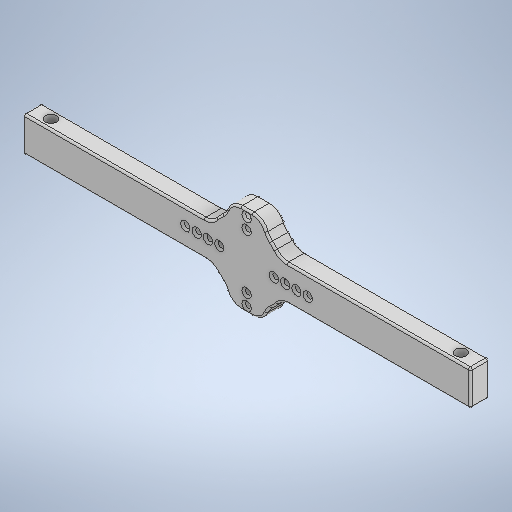
# Autodesk Inventor part: ServoAdapter
Saved by Autodesk Inventor 2025 (Build 290162000, 162)
## iProperties
Created: 2025-12-03
Part Number: ServoAdapter
Material: Generic
Document SubType Name: Modeling
Designer: ruven
Density: 1 g/cm^3
Appearance: Default
Author: ruven
Autodesk Inventor part; units mm, degrees
ref_plane "YZ Plane" through (0, 0, 0) normal (1, 0, 0) x (0, 1, 0)
ref_plane "XZ Plane" through (0, 0, 0) normal (0, 1, 0) x (-1, 0, 0)
ref_plane "XY Plane" through (0, 0, 0) normal (0, 0, 1) x (1, 0, 0)
sketch "Sketch1" plane through (0, 0, 0) normal (0, 1, 0) x (-1, 0, 0)
  line L0 (-59.4421, -4.3335) -> (-59.4421, 5)
  line L1 (59.4421, 4.3335) -> (59.4421, -5)
  line L2 (59.4421, -5) -> (-59.4421, 5) construction
  line L3 (-59.4421, -4.3335) -> (59.4421, 4.3335) construction
  line L4 (5, -59.443) -> (-5, -59.443)
  line L5 (-5, 59.443) -> (5, 59.443)
  line L6 (5, -59.443) -> (-5, 59.443) construction
  line L7 (-5, -59.443) -> (5, 59.443) construction
  circle A0 centre (0, 54.443) radius 2
  circle A1 centre (0, -54.443) radius 2
  line L8 (9.0122, 4.3335) -> (59.4421, 4.3335)
  line L9 (5, 18.5) -> (5, 8.6603)
  line L10 (5, 0.3645) -> (5, -0.4206)
  line L11 (5, -8.6603) -> (5, -18.5)
  line L12 (59.4421, -5) -> (8.6603, -5)
  line L13 (0.4206, -5) -> (-0.4206, -5)
  line L14 (-9.0122, -4.3335) -> (-59.4421, -4.3335)
  line L15 (-5, -18.5) -> (-5, -8.6603)
  line L16 (-5.0006, -0.3646) -> (-5.0006, 0.4206)
  line L17 (-5, 8.6603) -> (-5, 18.5)
  line L18 (-59.4421, 5) -> (-8.6603, 5)
  line L19 (-0.4206, 5) -> (0.4206, 5)
  circle A2 centre (0, 7.25) radius 0.75
  circle A3 centre (0, 10.25) radius 0.75
  circle A4 centre (0, 13.25) radius 0.75
  circle A5 centre (0, 16.25) radius 0.75
  line L20 (10.3146, 0) -> (-7.4821, 0) construction
  line L21 (0, -8.9076) -> (0, 6.1555) construction
  circle A6 centre (0, -7.25) radius 0.75
  circle A7 centre (0, -10.25) radius 0.75
  circle A8 centre (0, -13.25) radius 0.75
  circle A9 centre (0, -16.25) radius 0.75
  line L22 (59.443, -5) -> (-59.443, 5) construction
  line L23 (-5, -0.4206) -> (-5, 0.4206)
  circle A10 centre (-7.25, 0) radius 0.75
  circle A11 centre (-10.25, 0) radius 0.75
  circle A12 centre (-16.25, 0) radius 0.75
  circle A13 centre (-13.25, 0) radius 0.75
  line L24 (5, 0.4206) -> (5, -0.4206)
  circle A14 centre (7.25, 0) radius 0.75
  circle A15 centre (10.25, 0) radius 0.75
  circle A16 centre (13.25, 0) radius 0.75
  circle A17 centre (16.25, 0) radius 0.75
  line L25 (8.9076, 0) -> (-6.1555, 0) construction
  arc A18 (-0.7496, 10.2256) -> (-0.8594, 10.217) centre (0, 0) ccw
  arc A19 (0.8594, 10.217) -> (0.7496, 10.2256) centre (0, 0) ccw
  arc A20 (-5, 8.6603) -> (-8.6603, 5) centre (0, 0) ccw
  arc A21 (-10.217, 0.8594) -> (-10.2256, 0.7496) centre (0, 0) ccw
  arc A22 (-10.2258, -0.7496) -> (-10.2261, -0.7455) centre (0, 0) ccw
  arc A23 (-9.0122, -4.3335) -> (-5, -8.6603) centre (0, 0) ccw
  arc A24 (-0.8594, -10.217) -> (-0.7496, -10.2256) centre (0, 0) ccw
  arc A25 (0.7496, -10.2256) -> (0.8594, -10.217) centre (0, 0) ccw
  arc A26 (5, -8.6603) -> (8.6603, -5) centre (0, 0) ccw
  arc A27 (9.0122, 4.3335) -> (5, 8.6603) centre (0, 0) ccw
  arc A28 (10.217, -0.8594) -> (10.2256, -0.7496) centre (0, 0) ccw
  arc A29 (10.2532, 0) -> (10.2261, 0.7455) centre (0, 0) ccw
  line L26 (5, 18.5) -> (-5, 18.5)
  line L27 (-5, -18.5) -> (5, -18.5)
  point P0 (0, -59.443)
  point P1 (0, -6.1555)
  point P2 (6.1555, 0)
  point P3 (0, 0)
  dimension "d0" = 118.886
  dimension "d1" = 118.886
  dimension "d4" = 4
  dimension "d5" = 4
  dimension "d10" = 5
  dimension "d11" = 5
  dimension "d13" = 1.5
  dimension "d14" = 1.5
  dimension "d15" = 1.5
  dimension "d16" = 1.5
  dimension "d20" = 7.25
  dimension "d21" = 3
  dimension "d22" = 3
  dimension "d23" = 3
  dimension "d26" = 90
  dimension "d30" = 10
  dimension "d31" = 10
  dimension "d32" = 10
  dimension "d33" = 10
  dimension "d35" = 37
  dimension "d36" = 18.5
  constraints: 56 end point, 30 point on circle, 29 centre point, 20 parallel, 19 point on line, 8 perpendicular, 6 midpoint, 5 horizontal, 5 symmetric about line, 2 coincident, 1 vertical, 37 other
  measures "d0" distance of L0.end L1.start
  measures "d1" distance of L5.end L4.start
  measures "d4" diameter of A0
  measures "d5" diameter of A1
  measures "d10" distance from line of L5 A0.centre
  measures "d11" distance of point (0, -59.443) A1.centre
  measures "d13" diameter of A2
  measures "d14" diameter of A3
  measures "d15" diameter of A4
  measures "d16" diameter of A5
  measures "d20" distance of point (0, 0) A2.centre
  measures "d21" distance of A3.centre A2.centre
  measures "d22" distance of A4.centre A3.centre
  measures "d23" distance of A5.centre A4.centre
  measures "d30" radius of A27
  measures "d31" radius of A20
  measures "d32" radius of A23
  measures "d33" radius of A26
  measures "d35" distance between parallel lines of L27 L26
  measures "d36" distance from line of point (0, 0) L26
extrude "Extrusion1" add sketch "Sketch1" along normal blind 5 contours L0 L18 A22 A21 A11 L14 | A22 A11 A21 L18 A20 L17 A18 A3 A19 L9 A27 L8 A15 L12 A26 L11 A7 L15 A23 L14 | A22 A7 L11 L27 L15 | L17 L26 L9 A22 A19 A3 A18 | A22 A15 L8 L1 L12
sketch "Sketch2" plane through (0, 5, 0) normal (0, 1, 0) x (1, 0, 0)
  line L0 (-4.5, -18.5) -> (-5, -18.5) projected
  line L1 (-5, -18.5) -> (5.3219, -18.5)
  line L2 (5.3219, -18.5) -> (5.3219, -11.9)
  line L3 (5.3219, -11.9) -> (-5, -11.9)
  line L4 (-5, -11.9) -> (-5, -18.5)
  line L5 (-5, 18.5) -> (5.3219, 18.5)
  line L6 (5.3219, 18.5) -> (5.3219, 11.9)
  line L7 (5.3219, 11.9) -> (-5, 11.9)
  line L8 (-5, 11.9) -> (-5, 18.5)
  line L9 (5, 18.5) -> (-5, 18.5) projected
  point P0 (0, 0)
  point P1 (4.5, 18.5)
  point P2 (-4.5, 18.5)
  dimension "d37" = 6.6
  dimension "d38" = 6.6
  dimension "d39" = 0
  constraints: 16 end point, 4 parallel, 2 horizontal, 2 perpendicular, 2 point on line
  measures "d37" distance between parallel lines of L1 L3
  measures "d38" distance between parallel lines of L7 L5
  measures "d39" distance between parallel lines of L9 L5
extrude "Extrusion2" cut sketch "Sketch2" against normal through all
fillet "Fillet2" radius 4 12 edges at (5, 2.5, 11.9) (-5, 2.5, 11.9) (5, 2.5, -11.9) (-5, 2.5, -11.9) (9.0122, 2.5, -4.3335) (5, 2.5, -8.6603) (-5, 2.5, -8.6603) (-8.6603, 2.5, -5) (-9.0122, 2.5, 4.3335) (-5, 2.5, 8.6603) (5, 2.5, 8.6603) (8.6603, 2.5, 5)
fillet "Fillet3" radius 0.5 60 edges at (-6.5, 5, 0) (-3.7901, 0, 11.19) (3.7901, 0, 11.19) (-3.7901, 0, -11.19) (3.7901, 0, -11.19) (0, 0, 11.9) (7.0711, 0, 7.0711) (35.0829, 0, 5) (-35.3458, 0, 4.3335) (-7.2822, 0, 6.8534) (-3.7901, 5, 11.19) (3.7901, 5, 11.19) (-3.7901, 5, -11.19) (3.7901, 5, -11.19) (0, 5, 11.9) (7.0711, 5, 7.0711) (35.0829, 5, 5) (-35.3458, 5, 4.3335) (-7.2822, 5, 6.8534) (-35.0829, 0, -5) (0, 0, -11.9) (7.2822, 0, -6.8534) (35.3458, 0, -4.3335) (-7.0711, 0, -7.0711) (0.75, 5, -7.25) (0.75, 5, 10.25) (0.75, 5, -10.25) (-7.0711, 5, -7.0711) (-35.0829, 5, -5) (7.2822, 5, -6.8534) (35.3458, 5, -4.3335) (0, 5, -11.9) (11, 5, 0) (14, 5, 0) (59.4421, 2.5, -4.3335) (0.75, 5, 7.25) (-9.5, 5, 0) (-12.5, 5, 0) (-15.5, 5, 0) (-59.4421, 5, -0.3332) (59.4421, 5, 0.3332) (17, 5, 0) (8, 5, 0) (-59.4421, 2.5, 4.3335) (-59.4421, 0, -0.3332) (-59.4421, 2.5, -5) (59.4421, 0, 0.3332) (0.75, 0, -10.25) (17, 0, 0) (14, 0, 0) (11, 0, 0) (0.75, 0, -7.25) (-9.5, 0, 0) (-12.5, 0, 0) (-15.5, 0, 0) (8, 0, 0) (0.75, 0, 7.25) (0.75, 0, 10.25) (-6.5, 0, 0) (59.4421, 2.5, 5)
sketch "Sketch3" plane through (58.9421, 4.5, -4.3335) normal (0, 0, -1) x (-1, 0, 0)
  circle A0 centre (4.5, -2) radius 1.5
  line L0 (-0.5, 0) -> (-0.5, -4) projected
  line L1 (60.1921, 0.5) -> (57.6921, 0.5) projected
  line L2 (58.9421, 0.5) -> (58.9421, -4.5) construction
  circle A1 centre (113.3841, -2) radius 1.5
  point P0 (-0.5, -2)
  point P1 (58.4522, 0.5)
  point P2 (59.432, 0.5)
  dimension "d44" = 5
  dimension "d45" = 3
  constraints: 2 centre point, 2 end point, 2 midpoint, 1 symmetric about line, 1 vertical, 1 other
  measures "d44" distance of point (-0.5, -2) A0.centre
  measures "d45" diameter of A0
extrude "Extrusion3" cut sketch "Sketch3" along normal through all both and the other way through all
body "Solid1"
